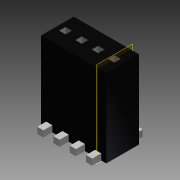
# Autodesk Inventor part: Recepticle_127
Saved by Autodesk Inventor 2014 (Build 180170000, 170)
## iProperties
Created: 2015-11-05
Part Number: Recepticle_127
Material: Generic
Document SubType Name: Modeling
Designer: Owner
Density: 1 g/cm^3
Appearance: Default
Author: Owner
Autodesk Inventor part; units mm, degrees
ref_plane "YZ Plane" through (0, 0, 0) normal (1, 0, 0) x (0, 1, 0)
ref_plane "XZ Plane" through (0, 0, 0) normal (0, 1, 0) x (-1, 0, 0)
ref_plane "XY Plane" through (0, 0, 0) normal (0, 0, 1) x (1, 0, 0)
sketch "Sketch1" plane through (0, 0, 0) normal (0, 1, 0) x (-1, 0, 0)
  line L0 (-2.1274, 0.9713) -> (2.9526, 0.9713)
  line L1 (2.9526, 0.9713) -> (2.9526, -1.5687)
  line L2 (2.9526, -1.5687) -> (-2.1274, -1.5687)
  line L3 (-2.1274, -1.5687) -> (-2.1274, 0.9713)
  point P0 (0, 0)
  dimension "d0" = 5.08
  dimension "d1" = 2.54
  constraints: 8 end point, 2 parallel, 1 horizontal, 1 perpendicular
  measures "d0" distance of L0.start L0.end
  measures "d1" distance of L0.end L1.end
extrude "Extrusion1" add sketch "Sketch1" along normal blind 6.1
ref_plane "Work Plane1" through (1.4924, 0, 0.9713) normal (1, 0, 0) x (0, 0, -1)
sketch "Sketch2" plane through (1.4924, 0, 0.9713) normal (1, 0, 0) x (0, 0, -1)
  line L0 (3.24, 0) -> (-0.7, 0)
  line L1 (-0.7, 0) -> (-0.7, 0.48)
  line L2 (-0.7, 0.48) -> (3.24, 0.48)
  line L3 (3.24, 0.48) -> (3.24, 0)
  line L4 (0, 0) -> (0, 6.1) projected
  point P0 (0.9713, 0)
  dimension "d5" = 3.94
  dimension "d6" = 0.7
  dimension "d7" = 0.48
  constraints: 8 end point, 2 parallel, 1 horizontal, 1 perpendicular
  measures "d5" distance of L0.start L0.end
  measures "d6" distance between parallel lines of L1 L4
  measures "d7" distance of L0.end L1.end
extrude "Extrusion2" add sketch "Sketch2" along normal mid plane 0.48
pattern_linear "Rectangular Pattern1" count 4 spacing 1.27 along (-1, 0, 0) of "Extrusion2"
sketch "Sketch3" plane through (0, 6.1, 0) normal (0, 1, 0) x (1, 0, 0)
  line L0 (2.1274, 1.5687) -> (-2.9526, 1.5687) projected
  line L1 (-2.9526, 1.5687) -> (-2.9526, -0.9713) projected
  line L2 (-2.5676, 0.5487) -> (-2.0676, 0.5487)
  line L3 (-2.0676, 0.5487) -> (-2.0676, 0.0487)
  line L4 (-2.0676, 0.0487) -> (-2.5676, 0.0487)
  line L5 (-2.5676, 0.0487) -> (-2.5676, 0.5487)
  point P0 (0, 0)
  dimension "d13" = 0.5
  dimension "d14" = 0.5
  dimension "d15" = 0.385
  dimension "d16" = 1.02
  constraints: 8 end point, 2 parallel, 1 horizontal, 1 perpendicular
  measures "d13" distance of L2.end L3.end
  measures "d14" distance of L2.start L2.end
  measures "d15" distance between parallel lines of L1 L5
  measures "d16" distance between parallel lines of L2 L0
extrude "Extrusion3" cut sketch "Sketch3" against normal through all
pattern_linear "Rectangular Pattern2" count 4 spacing 1.27 along (1, 0, 0) of "Extrusion3"
body "Solid1"
